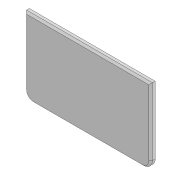
# Autodesk Inventor part: SlipersLåda 211018002
Saved by Autodesk Inventor 2020 (Build 240168000, 168)
## iProperties
Created: 2021-10-18
Part Number: SlipersLåda 211018002
Material: Generic
Document SubType Name: Modeling
Designer: dicpet001
Density: 1 g/cm^3
Appearance: Default
Author: dicpet001
Autodesk Inventor part; units mm, degrees
ref_plane "YZ Plane" through (0, 0, 0) normal (1, 0, 0) x (0, 1, 0)
ref_plane "XZ Plane" through (0, 0, 0) normal (0, 1, 0) x (-1, 0, 0)
ref_plane "XY Plane" through (0, 0, 0) normal (0, 0, 1) x (1, 0, 0)
sketch "Sketch1" plane through (0, 0, 0) normal (0, 0, 1) x (1, 0, 0)
  line L0 (0, 118.387) -> (0, -122.322) projected
  line L1 (-200.109, 0) -> (200.109, 0) projected
  line L2 (-139, 84) -> (139, 84)
  line L3 (139, 84) -> (139, -65)
  line L4 (120, -84) -> (-120, -84)
  line L5 (-139, -65) -> (-139, 84)
  arc A0 (-139, -65) -> (-120, -84) centre (-120, -65) ccw
  arc A1 (120, -84) -> (139, -65) centre (120, -65) ccw
  point P0 (0, 0)
  dimension "d0" = 278
  dimension "d1" = 168
  dimension "d2" = 19
  constraints: 8 end point, 4 point on circle, 4 tangent, 2 centre point, 2 parallel, 1 equal radius, 1 horizontal, 1 perpendicular, 2 other
  measures "d0" distance between parallel lines of L3 L5
  measures "d1" distance between parallel lines of L2 L4
  measures "d2" radius of A0
extrude "Extrusion1" add sketch "Sketch1" against normal blind 10
chamfer "Chamfer1" distance 4 angle 45 6 edges at (139, 9.5, 0) (133.435, -78.435, 0) (0, -84, 0) (-133.435, -78.435, 0) (-139, 9.5, 0) (0, 84, 0)
body "Solid1"
